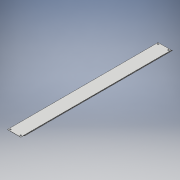
# Autodesk Inventor part: sideplate part 2 mirror
Saved by Autodesk Inventor 2018 (Build 220112000, 112)
## iProperties
Created: 2018-06-15
Part Number: sideplate part 2 mirror
Material: Generic
Document SubType Name: Sheet Metal
Designer: John Viljoen
Density: 1 g/cm^3
Sheet Metal Rule: Default_mm
Appearance: Default
Author: John Viljoen
Autodesk Inventor part; units mm, degrees
ref_plane "YZ Plane" through (0, 0, 0) normal (1, 0, 0) x (0, 1, 0)
ref_plane "XZ Plane" through (0, 0, 0) normal (0, 1, 0) x (-1, 0, 0)
ref_plane "XY Plane" through (0, 0, 0) normal (0, 0, 1) x (1, 0, 0)
sketch "Sketch1" plane through (0, 0, 0) normal (0, 0, 1) x (1, 0, 0)
  line L0 (0, 0) -> (29.621, 0)
  line L1 (29.621, 0) -> (29.621, 338.525)
  line L2 (29.621, 338.525) -> (0, 338.525)
  line L3 (0, 338.525) -> (0, 0)
  dimension "d0" = 29.621
  dimension "d1" = 338.525
  measures "d0" distance of L2.end L1.end
  measures "d1" distance of L1.end L0.end
extrude "Plate1" add sketch "Sketch1" along normal blind 0.5
sketch "Sketch2" plane through (30.1974, 338.525, 0.6152) normal (0.3842953, 0, -0.9232102) x (0, 1, 0)
  line L0 (-338.525, 0) -> (0, 0)
  line L1 (0, 0) -> (0, 2.0004)
  line L2 (0, 2.0004) -> (-338.525, 2.0004)
  line L3 (-338.525, 2.0004) -> (-338.525, 0)
  constraints: 6 end point, 1 horizontal, 1 perpendicular, 1 vertical
edge flange "Flange1" height 2.4 angle 22.6 thickness 0.5 bend radius 1.5 thickness toward (0.3842953, 0, -0.9232102) relief straight relief width 0.5 relief depth 0.25 edges at (29.621, 169.2625, 0.5) wall of the first edge with corners at (30.1974, 0, 0.6152) (30.1974, 338.525, 0.6152) (32.0442, 338.525, 1.3839) (32.0442, 0, 1.3839)
bend "Bend1"
corner "Corner1"
sketch "Sketch3" plane through (0, 0, 0) normal (0, 0, -1) x (-1, 0, 0)
  line L0 (0, 0) -> (-55.5693, 0)
  line L1 (-55.5693, 0) -> (-55.5693, 6.35)
  line L2 (-55.5693, 6.35) -> (0, 6.35)
  line L3 (0, 6.35) -> (0, 0)
  dimension "d13" = 6.35
  constraints: 8 end point, 2 parallel, 1 horizontal, 1 perpendicular
  measures "d13" distance of L0.end L1.end
extrude "Extrusion1" cut sketch "Sketch3" against normal blind 10
sketch "Sketch4" plane through (0, 0, 0) normal (0, 0, -1) x (-1, 0, 0)
  line L0 (0, 6.35) -> (-29.621, 6.35)
  line L1 (-29.621, 6.35) -> (-29.621, 0)
  line L2 (-29.621, 0) -> (0, 0)
  line L3 (0, 0) -> (0, 6.35)
  constraints: 8 end point, 2 parallel, 1 horizontal, 1 perpendicular
extrude "Extrusion2" add sketch "Sketch4" against normal up to surface (0.5 mm away)
sketch "Sketch5" plane through (0, 0, 0.5) normal (0, 0, 1) x (1, 0, 0)
  line L0 (29.621, 6.35) -> (29.621, 0) projected
  line L1 (0, 0) -> (0, 3.175) construction
  line L2 (0, 0) -> (0, 338.525) construction
  line L3 (0, 3.175) -> (3.175, 3.175) construction
  line L4 (29.621, 0) -> (29.621, 3.175) construction
  line L5 (29.621, 3.175) -> (26.446, 3.175) construction
  circle A0 centre (3.175, 3.175) radius 1.5
  circle A1 centre (26.446, 3.175) radius 1.5
  dimension "d18" = 3.175
  dimension "d19" = 3.175
  dimension "d20" = 3.175
  dimension "d21" = 3.175
  dimension "d22" = 3
  dimension "d23" = 3
  constraints: 8 end point, 2 centre point, 2 coincident, 2 perpendicular, 1 midpoint, 1 point on line
  measures "d18" distance of L1.start L1.end
  measures "d19" distance of L1.end L3.end
  measures "d20" distance of L0.end L4.end
  measures "d21" distance of L4.end L5.end
  measures "d22" diameter of A0
  measures "d23" diameter of A1
extrude "Extrusion3" cut sketch "Sketch5" against normal blind 10
sketch "Sketch6" plane through (0, 0, 0.5) normal (0, 0, 1) x (1, 0, 0)
  line L0 (0, 338.525) -> (0, 335.35) construction
  line L1 (0, 0) -> (0, 338.525) construction
  line L2 (0, 335.35) -> (3.175, 335.35) construction
  line L3 (29.621, 338.525) -> (29.621, 335.35) construction
  line L4 (29.621, 6.35) -> (29.621, 338.525) construction
  line L5 (29.621, 335.35) -> (26.446, 335.35) construction
  circle A0 centre (3.175, 335.35) radius 1.5
  circle A1 centre (26.446, 335.35) radius 1.5
  dimension "d26" = 3.175
  dimension "d27" = 3.175
  dimension "d28" = 3.175
  dimension "d29" = 3.175
  dimension "d30" = 3
  dimension "d31" = 3
  constraints: 8 end point, 2 centre point, 2 coincident, 2 point on line, 1 horizontal, 1 perpendicular
  measures "d26" distance of L0.start L0.end
  measures "d27" distance of L0.end L2.end
  measures "d28" distance of L3.start L3.end
  measures "d29" distance of L3.end L5.end
  measures "d30" diameter of A0
  measures "d31" diameter of A1
extrude "Extrusion4" cut sketch "Sketch6" against normal blind 10
equation "\"d2\" = Thickness"
equation "\"d3\" = BendReliefWidth"
equation "\"d4\" = BendReliefDepth"
equation "\"d5\" = MinimumRemnant"
equation "\"d6\" = TransitionRadius"
equation "\"d10\" = CornerReliefSize"
equation "\"d11\" = GapSize"
equation "\"d12\" = JacobiRadiusSize"
equation "\"BendRadius\" = Thickness"
equation "\"BendReliefWidth\" = Thickness"
equation "\"BendReliefDepth\" = 0.5 * Thickness"
equation "\"CornerReliefSize\" = 4 * Thickness"
equation "\"MinimumRemnant\" = 2 * Thickness"
equation "\"TransitionRadius\" = BendRadius"
equation "\"JacobiRadiusSize\" = BendRadius"
equation "\"GapSize\" = Thickness"
equation "\"Thickness\" = 0.5"
body "Solid1"
